Autodesk Fusion 360 part; units mm, degrees
note: some values were not read from the file. Set by a fixed rule: which sketch regions a step uses.
(part 3 of 3)
sketch "Sketch1 (2)" plane through (0, 0, 0) normal (0, 0, 1) x (1, 0, 0) in component "Legs"
  line L0 (15.0415, 14.9314) -> (-14.9585, 14.9314)
  line L1 (-14.9585, 14.9314) -> (-14.9585, -15.0686)
  line L2 (-14.9585, -15.0686) -> (15.0415, -15.0686)
  line L3 (15.0415, -15.0686) -> (15.0415, 14.9314)
  line L4 (15.0415, 14.9314) -> (-14.9585, -15.0686) construction
  line L5 (-14.9585, 14.9314) -> (15.0415, -15.0686) construction
  line L6 (0.0415, 14.9314) -> (0.0415, -15.0686) construction
  line L7 (-14.9585, -0.0686) -> (15.0415, -0.0686) construction
  point P0 (0.0415, -0.0686)
  dimension "d80" = 30
  dimension "d81" = 30
  constraint horizontal L0
  constraint perpendicular L0 L1
  constraint parallel L0 L2
  constraint parallel L1 L3
  constraint coincident L4 P0
  constraint coincident L5 P0
  constraint midpoint L0 L6.start
  constraint midpoint L2 L6.end
  constraint midpoint L1 L7.start
  constraint midpoint L3 L7.end
  measures "d80" distance of L1.end L2.end
  measures "d81" distance of L0.end L1.end
extrude "Extrude1'" [suppressed] in component "Lid"
extrude "Extrude2'" [suppressed] in component "Lid"
extrude "Extrude3'" [suppressed] in component "Lid"
extrude "Extrude4" [suppressed] in component "Lid"
extrude "Extrude5" [suppressed] in component "Lid"
extrude "Extrude6" [suppressed] in component "Lid"
extrude "Extrude7" [suppressed] in component "Lid"
extrude "Extrude8'" [suppressed] in component "Lid"
extrude "Extrude9'" [suppressed] in component "Lid"
extrude "Extrude1''" [suppressed]
extrude "Extrude4'" [suppressed]
combine "Combine1" [suppressed]
extrude "Extrude3''" [suppressed]
extrude "Extrude2''" [suppressed]
component "Base" placed x (1, 0, 0) y (0, 1, 0) z (0, 0, 1) at (0, 0, 0)
component "Lid" placed x (1, 0, 0) y (0, 1, 0) z (0, 0, 1) at (0, 0, 0)
component "Legs" placed x (1, 0, 0) y (0, 1, 0) z (0, 0, 1) at (0, 0, 0)
